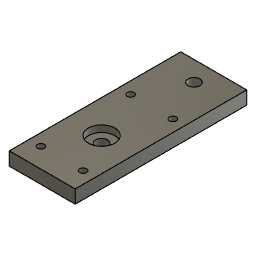
TEST (v12~recovered) v1 (Autodesk Fusion 360 design; units mm, degrees)
Autodesk Fusion 360 part; units mm, degrees
sketch "Esquisse1" plane through (0, 0, 0) normal (0, 1, 0) x (1, 0, 0)
  line L0 (0, 0) -> (50, 0)
  line L1 (50, 0) -> (50, 130)
  line L2 (50, 130) -> (0, 130)
  line L3 (0, 130) -> (0, 0)
  circle A0 centre (25, 45) radius 4.5
  circle A1 centre (25, 115) radius 4.5
  circle A2 centre (9, 83) radius 2.6
  circle A3 centre (41, 83) radius 2.6
  circle A4 centre (9, 15) radius 2.6
  circle A5 centre (41, 15) radius 2.6
  dimension "d1" = 50
  dimension "d2" = 130
  dimension "d3" = 9
  dimension "d4" = 9
  dimension "d5" = 5.2
  dimension "d6" = 5.2
  dimension "d7" = 5.2
  dimension "d8" = 5.2
  dimension "d9" = 25
  dimension "d10" = 25
  dimension "d11" = 15
  dimension "d12" = 15
  dimension "d13" = 30
  dimension "d14" = 15
  dimension "d15" = 32
  dimension "d16" = 32
  dimension "d17" = 32
  dimension "d18" = 32
  dimension "d19" = 9
  dimension "d20" = 9
  constraint horizontal L0
  constraint vertical L1
  constraint horizontal L2
  constraint vertical L3
  constraint coincident L0.start L3.end
  measures "d1" distance of L0.start L0.end
  measures "d2" distance of L0.start L2.end
  measures "d3" diameter of A0
  measures "d4" diameter of A1
  measures "d5" diameter of A2
  measures "d6" diameter of A3
  measures "d7" diameter of A4
  measures "d8" diameter of A5
  measures "d9" distance of L3 A1.centre
  measures "d10" distance of L3 A0.centre
  measures "d11" distance of L0 A4.centre
  measures "d12" distance of L0 A5.centre
  measures "d13" vertical distance of A0.centre A4.centre
  measures "d14" distance of L2 A1.centre
  measures "d15" vertical distance of A1.centre A2.centre
  measures "d16" vertical distance of A1.centre A3.centre
  measures "d17" distance of A4.centre A5.centre
  measures "d18" distance of A2.centre A3.centre
  measures "d19" distance of L3 A2.centre
  measures "d20" distance of L3 A4.centre
extrude "Extrusion2" add sketch "Esquisse1" along normal blind 10
sketch "Esquisse7" plane through (0, 10, 0) normal (0, 1, 0) x (-1, 0, 0)
  circle A0 centre (-41, -15) radius 2.6
  circle A1 centre (-9, -15) radius 2.6
  circle A2 centre (-41, -83) radius 2.6
  circle A3 centre (-9, -83) radius 2.6
  circle A4 centre (-25, -115) radius 4.5
  circle A5 centre (-25, -45) radius 4.5
  line L0 (0, -130) -> (0, 0)
  line L1 (0, 0) -> (-50, 0)
  line L2 (-50, 0) -> (-50, -130)
  line L3 (-50, -130) -> (0, -130)
  circle A6 centre (-25, -45) radius 10
  dimension "d28" = 20
  constraint concentric A5 A6
  measures "d28" diameter of A6
extrude "Extrusion3" cut sketch "Esquisse7" against normal blind 5 contours A6
